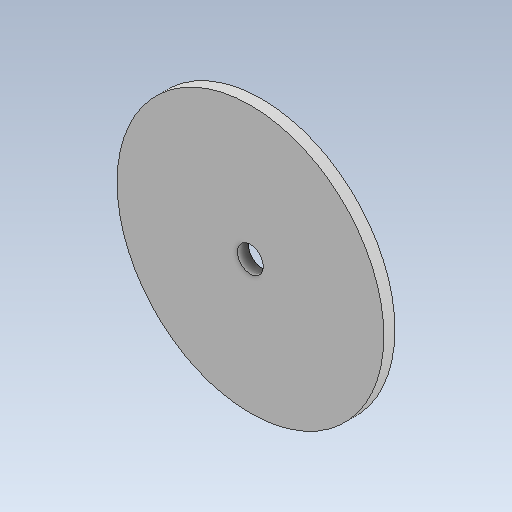
# Autodesk Inventor part: SealV3
Saved by Autodesk Inventor 2020 (Build 240168000, 168)
## iProperties
Created: 2020-04-09
Part Number: SealV3
Material: Generic
Document SubType Name: Modeling
Designer: Theo Cominotto
Density: 1 g/cm^3
Appearance: Default
Author: Theo Cominotto
Autodesk Inventor part; units mm, degrees
ref_plane "YZ Plane" through (0, 0, 0) normal (1, 0, 0) x (0, 1, 0)
ref_plane "XZ Plane" through (0, 0, 0) normal (0, 1, 0) x (-1, 0, 0)
ref_plane "XY Plane" through (0, 0, 0) normal (0, 0, 1) x (1, 0, 0)
sketch "Sketch1" plane through (0, 0, 0) normal (0, 0, 1) x (1, 0, 0)
  circle A0 centre (0, 0) radius 18
  circle A1 centre (0, 0) radius 1.75
  dimension "d0" = 36
  dimension "d1" = 3.5
  constraints: 2 centre point, 2 coincident
  measures "d0" diameter of A0
  measures "d1" diameter of A1
extrude "Extrusion1" add sketch "Sketch1" along normal blind 1.5
equation "\"d2\" = 0.5 * platformT"
equation "\"TaperEnd\" = 22"
equation "\"TaperStart\" = 22.5"
equation "\"sealD\" = 12.5"
equation "\"WallT\" = 1.6"
equation "\"platformT\" = 3"
equation "\"ThreadPitch\" = 1.5"
equation "\"ThreadMajor\" = TaperStart + 2 * ThreadHeight"
equation "\"ThreadTol\" = 0.32"
equation "\"SpringPin\" = 6.6"
equation "\"ThreadHeight\" = 0.6"
body "Solid1"
